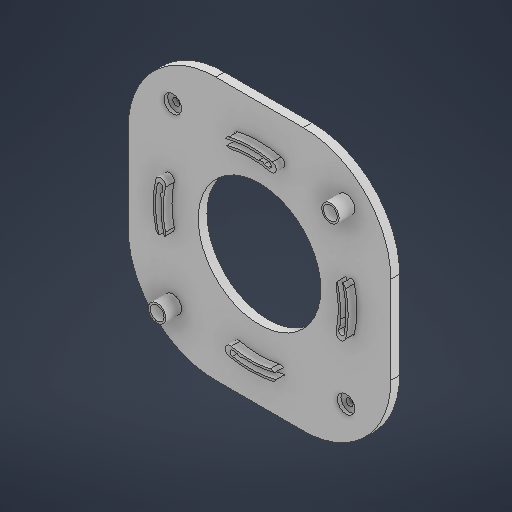
# Autodesk Inventor part: Female plug&play
Saved by Autodesk Inventor 2026.1 (Build 301233000, 233)
## iProperties
Created: 2026-03-06
Part Number: Female plug&play
Material: Generic
Document SubType Name: Modeling
Designer: Kevin's Nabil
Density: 1 g/cm^3
Appearance: Default
Author: Kevin's Nabil
Autodesk Inventor part; units mm, degrees
ref_plane "YZ Plane" through (0, 0, 0) normal (1, 0, 0) x (0, 1, 0)
ref_plane "XZ Plane" through (0, 0, 0) normal (0, 1, 0) x (-1, 0, 0)
ref_plane "XY Plane" through (0, 0, 0) normal (0, 0, 1) x (1, 0, 0)
sketch "Sketch1" plane through (0, 0, 0) normal (0, 0, 1) x (1, 0, 0)
  line L0 (-75, -75) -> (75, -75)
  line L1 (75, -75) -> (75, 75)
  line L2 (75, 75) -> (-75, 75)
  line L3 (-75, 75) -> (-75, -75)
  line L4 (-75, -75) -> (75, 75) construction
  line L5 (75, -75) -> (-75, 75) construction
  arc A0 (51.4783, -11.796) -> (51.4817, 11.7813) centre (0, 0) ccw
  arc A1 (53.3699, -10.5361) -> (53.3699, 10.5361) centre (0, 0) ccw
  arc A2 (50.2551, -9.9212) -> (50.2551, 9.9212) centre (0, 0) ccw
  arc A3 (53.3699, 10.5361) -> (50.2551, 9.9212) centre (51.8125, 10.2286) ccw
  arc A4 (50.2551, -9.9212) -> (53.3699, -10.5361) centre (51.8096, -10.2434) ccw
  line L6 (0, 0) -> (120.3079, 0)
  spline S0 degree 2 poles (51.0287, -4.4801) (52.1004, -7.1283) (50.6557, -7.6159) knots 0 0 0 1 1 1
  arc A5 (54.2233, -12.4087) -> (54.2233, 12.4087) centre (0, 0) ccw
  arc A6 (48.74, -11.1539) -> (48.74, 11.1539) centre (0, 0) ccw
  arc A7 (54.2233, 12.4087) -> (48.74, 11.1539) centre (51.4817, 11.7813) ccw
  arc A8 (48.74, -11.1539) -> (54.2233, -12.4087) centre (51.4817, -11.7813) ccw
  arc A9 (53.3639, -10.5665) -> (52.4539, 14.4204) centre (0, 0) ccw
  arc A10 (50.2494, -9.9498) -> (49.3745, 13.6441) centre (0, 0) ccw
  circle A11 centre (49.4975, 49.4975) radius 5
  circle A12 centre (-49.4975, -49.4975) radius 5
  circle A13 centre (49.4975, 49.4975) radius 4
  circle A14 centre (-49.4975, -49.4975) radius 4
  point P0 (52.8125, 0)
  point P1 (28.5375, -29.3076)
  point P2 (51.5021, -11.8009)
  point P3 (51.4042, -6.894)
  point P4 (53.3699, 10.5361)
  point P5 (50.2551, 9.9212)
  dimension "d0" = 150
  dimension "d1" = 150
  dimension "d2" = 52.8125
  dimension "d6" = 102.45
  dimension "d7" = 108.8
  dimension "d8" = 4.185
  dimension "d12" = 111.25
  dimension "d13" = 100
  dimension "d21" = 10
  dimension "d22" = 10
  dimension "d23" = 8
  dimension "d24" = 8
  dimension "d39" = 70
  dimension "d40" = 70
  constraints: 33 point on circle, 15 centre point, 14 coincident, 14 end point, 3 symmetric about line, 2 horizontal, 2 midpoint, 2 parallel, 2 tangent, 1 perpendicular, 1 point on line, 4 other
  measures "d0" distance of L2.end L1.end
  measures "d1" distance of L1.end L0.end
  measures "d2" distance of point (0, 0) point (52.812, 0)
  measures "d6" diameter of A2
  measures "d7" diameter of A1
  measures "d8" vertical distance of point (51.502, -11.801) point (50.656, -7.616)
  measures "d12" diameter of A5
  measures "d13" diameter of A6
  measures "d21" diameter of A11
  measures "d22" diameter of A12
  measures "d23" diameter of A13
  measures "d24" diameter of A14
  measures "d39" distance of point (0, 0) A11.centre
  measures "d40" distance of point (0, 0) A12.centre
extrude "Extrusion1" add sketch "Sketch1" against normal blind 5 contours A5 A8 A6 L6 A2 A4 A1 | L6 A1 A9 A7 A5 | L3 L2 L1 L0 | L6 A0 A3 A1 | A1 A4 A0 L6 | A3 A10 A7 A9 | L6 A2 A3 A0 | A0 A4 A2 S0 L6 | L6 A6 A7 A10 A2 | S0 A2 | A11 | A12 | A13 | A14
extrude "Extrusion2" add sketch "Sketch1" along normal blind 5 contours A5 A8 A6 L6 A2 A4 A1 | L6 A1 A9 A7 A5 | L6 A6 A7 A10 A2 | S0 A2
pattern_circular "Circular Pattern1" count 4 over 360 about axis through (0, 0, -10) along (0, 0, 1) of "Extrusion2"
extrude "Extrusion4" add sketch "Sketch1" along normal blind 9 contours A11 | A12
extrude "Extrusion5" cut sketch "Sketch1" against normal through all contours A13 | A14
fillet "Fillet1" radius 50 4 edges at (-75, 75, -2.5) (75, 75, -2.5) (75, -75, -2.5) (-75, -75, -2.5)
sketch "Sketch3" plane through (0, 0, 0) normal (0, 0, 1) x (1, 0, 0)
  circle A0 centre (0, 0) radius 35
  circle A1 centre (49.4975, 49.4975) radius 5 projected
  line L0 (-49.4975, -49.4975) -> (49.4975, 49.4975) construction
  line L1 (49.4975, -49.4975) -> (-49.4975, 49.4975) construction
  circle A2 centre (-49.4975, 49.4975) radius 2.05
  circle A3 centre (49.4975, -49.4975) radius 2.05
  circle A4 centre (-49.4975, 49.4975) radius 5
  circle A5 centre (49.4975, -49.4975) radius 5
  dimension "d30" = 70
  dimension "d31" = 4.1
  dimension "d32" = 4.1
  dimension "d33" = 10
  dimension "d34" = 10
  dimension "d41" = 70
  constraints: 5 centre point, 5 coincident, 4 end point, 2 midpoint
  measures "d30" diameter of A0
  measures "d31" diameter of A2
  measures "d32" diameter of A3
  measures "d33" diameter of A4
  measures "d34" diameter of A5
  measures "d41" distance of point (0, 0) L1.end
extrude "Extrusion6" cut sketch "Sketch3" against normal through all contours A0 | A2 | A3
extrude "Extrusion7" cut sketch "Sketch3" against normal blind 2 contours A3 | A4 | A5
equation "\"d22\" = d21"
equation "\"d24\" = d23"
equation "\"d40\" = d39"
body "Solid1"
